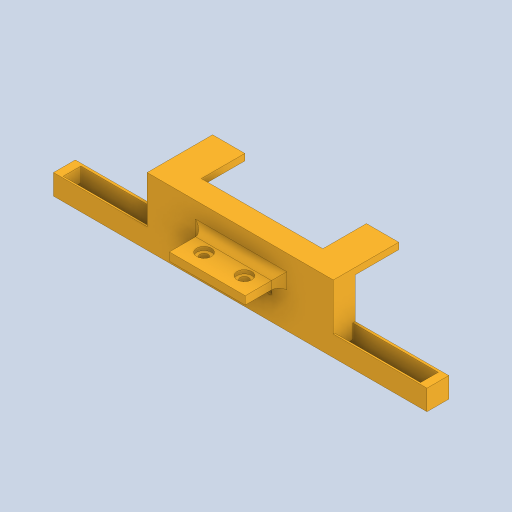
# Autodesk Inventor part: konsept3_med_led_extended
Saved by Autodesk Inventor 2023.1 (Build 271208000, 208)
## iProperties
Created: 2024-07-10
Part Number: konsept3_med_led_extended
Material: S355J2+N
Document SubType Name: Modeling
Designer: huchonms
Engineer: thingelstade
Mass: 592.93 g
Surface Area: 269.172 cm^2
Volume: 75.5325 cm^3
Density: 7.85 g/cm^3
Appearance: Metal (300-500 MPa)
tc_part_rev_length: 231
tc_part_rev_width: 62
tc_part_rev_height: 41.64
tc_part_rev_uom_length: mm
tc_part_rev_volume: 75533
tc_part_rev_uom_volume: mm^3
tc_part_rev_mass: 0.59
tc_part_rev_uom_mass: kg
NOV_FileName: konsept3_med_led_extended
Author: huchonms
Revision Number: 0
Autodesk Inventor part; units mm, degrees
ref_plane "YZ Plane" through (0, 0, 0) normal (1, 0, 0) x (0, 1, 0)
ref_plane "XZ Plane" through (0, 0, 0) normal (0, 1, 0) x (-1, 0, 0)
ref_plane "XY Plane" through (0, 0, 0) normal (0, 0, 1) x (1, 0, 0)
sketch "Sketch1" plane through (0, 0, 0) normal (0, 1, 0) x (-1, 0, 0)
  circle A0 centre (74.3729, -21.8037) radius 1.7645
  circle A1 centre (56.3729, -21.8037) radius 3.0578
  circle A2 centre (38.3729, -21.8037) radius 1.7645
  ellipse E0 centre (18.2576, -20.2741) end of major axis (25.2624, -10.1128) minor radius 8.7701 (8.7502, -27.1013) -> (10.9663, -30.2256) ccw
  spline S0 degree 3 poles (10.9663, -30.2256) (11.558, -30.6853) (12.2409, -31.0443) (12.9908, -31.2838) (13.7407, -31.5232) (14.557, -31.6429) (15.405, -31.6429) knots 0 0 0 0 0.499989 0.499989 0.499989 1 1 1 1
  line L0 (15.405, -31.6429) -> (97.3407, -31.6429)
  spline S1 degree 3 poles (97.3407, -31.6429) (98.1082, -31.6429) (98.8584, -31.5451) (99.5616, -31.3425) (100.2492, -31.1443) (100.8915, -30.8461) (101.4652, -30.4546) (102.0389, -30.063) (102.5439, -29.5783) (102.9657, -29.0193) (103.3971, -28.4476) (103.7414, -27.7985) (103.9955, -27.1013) knots 2.676287 2.676287 2.676287 2.676287 2.891386 2.891386 2.891386 3.101723 3.101723 3.101723 3.312059 3.312059 3.312059 3.527157 3.527157 3.527157 3.527157
  line L1 (103.9955, -27.1013) -> (111.6432, -6.1177)
  spline S2 degree 3 poles (111.6432, -6.1177) (111.7397, -5.8528) (111.8344, -5.5944) (112.022, -5.0857) (112.1147, -4.8357) (112.3029, -4.3319) (112.398, -4.0794) (112.5844, -3.5887) (112.6755, -3.351) (112.8621, -2.8692) (112.9568, -2.6278) (113.1123, -2.2368) (113.1754, -2.0801) (113.2982, -1.7787) (113.3578, -1.6344) (113.4677, -1.3725) (113.5183, -1.2539) (113.6125, -1.0372) (113.6562, -0.9386) (113.7358, -0.763) (113.772, -0.685) (113.8392, -0.544) (113.8704, -0.4806) (113.9275, -0.3682) (113.9537, -0.3186) (113.9875, -0.2575) (113.9966, -0.2414) (114.0055, -0.226) knots 5.498338 5.498338 5.498338 5.498338 5.552114 5.552114 5.607126 5.607126 5.666519 5.666519 5.727103 5.727103 5.795218 5.795218 5.844696 5.844696 5.895721 5.895721 5.943374 5.943374 5.988975 5.988975 6.031119 6.031119 6.071863 6.071863 6.110843 6.110843 6.125778 6.125778 6.125778 6.125778
  spline S3 degree 3 poles (114.0055, -0.226) (113.9928, -0.2026) (113.9622, -0.1742) (113.9104, -0.1385) (113.906, -0.1355) (113.8757, -0.1152) (113.8463, -0.0979) (113.8052, -0.0766) (113.7959, -0.0719) (113.691, -0.0221) (113.6027, 0) (113.5195, 0) knots 0 0 0 0 0.234375 0.234375 0.25 0.25 0.4375 0.4375 0.5 0.5 0.999999 0.999999 0.999999 0.999999
  line L2 (112.7702, 0) -> (113.5195, 0)
  line L3 (112.7702, 0) -> (112.7455, 0)
  line L4 (0, 0) -> (112.7455, 0)
  line L5 (0, 0) -> (-0.0247, 0)
  line L6 (-0.7737, 0) -> (-0.0247, 0)
  spline S4 degree 3 poles (-0.7737, 0) (-0.846, 0) (-0.9227, -0.017) (-1.0154, -0.0558) (-1.0288, -0.0618) (-1.0767, -0.0844) (-1.1139, -0.1052) (-1.153, -0.1307) (-1.1545, -0.1317) (-1.2121, -0.1699) (-1.246, -0.2006) (-1.2597, -0.226) knots 0.000001 0.000001 0.000001 0.000001 0.4375 0.4375 0.5 0.5 0.734375 0.734375 0.75 0.75 1 1 1 1
  spline S5 degree 3 poles (-1.2597, -0.226) (-1.2124, -0.3083) (-1.1576, -0.413) (-1.0955, -0.5406) (-0.951, -0.8374) (-0.7663, -1.2588) (-0.545, -1.7976) (-0.5269, -1.8415) (-0.5086, -1.8863) (-0.4901, -1.9318) (-0.0669, -2.9705) (0.4808, -4.4117) (1.1025, -6.1177) knots 3.299 3.299 3.299 3.299 3.378966 3.378966 3.378966 3.564913 3.564913 3.564913 3.580082 3.580082 3.580082 3.92644 3.92644 3.92644 3.92644
  line L7 (1.1025, -6.1177) -> (8.7502, -27.1013)
  circle A3 centre (56.3729, -21.8037) radius 3.0578
  circle A4 centre (38.3729, -21.8037) radius 1.7645
  circle A5 centre (74.3729, -21.8037) radius 1.7645
  point P0 (47.4044, 14.458)
  constraints: 16 end point, 6 centre point, 17 other
extrude "Extrusion1" add sketch "Sketch1" along normal blind 7.5
sketch "Sketch3" plane through (0, 0, 0) normal (0, 1, 0) x (-1, 0, 0)
  line L0 (32.2898, -10.7134) -> (79.2898, -10.7134)
  line L1 (79.2898, -10.7134) -> (79.2898, -15.7134)
  line L2 (79.2898, -15.7134) -> (32.2898, -15.7134)
  line L3 (32.2898, -15.7134) -> (32.2898, -10.7134)
  point P0 (0, 0)
  constraints: 8 end point, 2 parallel, 1 horizontal, 1 perpendicular
extrude "Extrusion2" add sketch "Sketch3" against normal blind 21
sketch "Sketch4" plane through (0, 0, 0) normal (0, -1, 0) x (1, 0, 0)
  circle A0 centre (-56.3729, -21.8037) radius 3.0578 projected
  circle A1 centre (-56.3729, -21.8037) radius 6.1
  point P0 (0, 0)
  dimension "d6" = 12.2
  constraints: 1 centre point, 1 coincident
  measures "d6" diameter of A1
extrude "Extrusion3" cut sketch "Sketch4" against normal blind 3.5
sketch "Sketch5" plane through (0, 7.5, 0) normal (0, 1, 0) x (1, 0, 0)
  spline S0 degree 3 poles (1.2597, 0.226) (1.2124, 0.3083) (1.1576, 0.413) (1.0955, 0.5406) (0.951, 0.8374) (0.7663, 1.2588) (0.545, 1.7976) (0.5269, 1.8415) (0.5086, 1.8863) (0.4901, 1.9318) (0.0669, 2.9705) (-0.4808, 4.4117) (-1.1025, 6.1177) knots 0 0 0 0 0.127447 0.127447 0.127447 0.423807 0.423807 0.423807 0.447982 0.447982 0.447982 1 1 1 1 projected
  line L0 (-1.1025, 6.1177) -> (-8.7502, 27.1013) projected
  ellipse E0 centre (-18.2576, 20.2741) end of major axis (-25.2624, 10.1128) minor radius 8.7701 (-8.7502, 27.1013) -> (-10.9663, 30.2256) ccw projected
  spline S1 degree 3 poles (-10.9663, 30.2256) (-11.558, 30.6853) (-12.2409, 31.0443) (-12.9908, 31.2838) (-13.7407, 31.5232) (-14.557, 31.6429) (-15.405, 31.6429) knots 0 0 0 0 0.499989 0.499989 0.499989 1 1 1 1 projected
  line L1 (-15.405, 31.6429) -> (-97.3407, 31.6429) projected
  spline S2 degree 3 poles (-97.3407, 31.6429) (-98.1082, 31.6429) (-98.8584, 31.5451) (-99.5616, 31.3425) (-100.2492, 31.1443) (-100.8915, 30.8461) (-101.4652, 30.4546) (-102.0389, 30.063) (-102.5439, 29.5783) (-102.9657, 29.0193) (-103.3971, 28.4476) (-103.7414, 27.7985) (-103.9955, 27.1013) knots 0 0 0 0 0.252799 0.252799 0.252799 0.500001 0.500001 0.500001 0.747202 0.747202 0.747202 1 1 1 1 projected
  line L2 (-103.9955, 27.1013) -> (-111.6432, 6.1177) projected
  spline S3 degree 3 poles (-111.6432, 6.1177) (-111.7397, 5.8528) (-111.8344, 5.5944) (-112.022, 5.0857) (-112.1147, 4.8357) (-112.3029, 4.3319) (-112.398, 4.0794) (-112.5844, 3.5887) (-112.6755, 3.351) (-112.8621, 2.8692) (-112.9568, 2.6278) (-113.1123, 2.2368) (-113.1754, 2.0801) (-113.2982, 1.7787) (-113.3578, 1.6344) (-113.4677, 1.3725) (-113.5183, 1.2539) (-113.6125, 1.0372) (-113.6562, 0.9386) (-113.7358, 0.763) (-113.772, 0.685) (-113.8392, 0.544) (-113.8704, 0.4806) (-113.9275, 0.3682) (-113.9537, 0.3186) (-113.9875, 0.2575) (-113.9966, 0.2414) (-114.0055, 0.226) knots 0 0 0 0 0.085707 0.085707 0.173384 0.173384 0.268043 0.268043 0.364601 0.364601 0.473161 0.473161 0.552018 0.552018 0.633341 0.633341 0.709288 0.709288 0.781966 0.781966 0.849134 0.849134 0.914072 0.914072 0.976197 0.976197 1 1 1 1 projected
  spline S4 degree 3 poles (-114.0055, 0.226) (-113.9928, 0.2026) (-113.9622, 0.1742) (-113.9104, 0.1385) (-113.906, 0.1355) (-113.8757, 0.1152) (-113.8463, 0.0979) (-113.8052, 0.0766) (-113.7959, 0.0719) (-113.691, 0.0221) (-113.6027, 0) (-113.5195, 0) knots 0 0 0 0 0.234375 0.234375 0.25 0.25 0.4375 0.4375 0.5 0.5 1 1 1 1 projected
  line L3 (-113.5195, 0) -> (0.7737, 0) projected
  spline S5 degree 3 poles (0.7737, 0) (0.846, 0) (0.9227, 0.017) (1.0154, 0.0558) (1.0288, 0.0618) (1.0767, 0.0844) (1.1139, 0.1052) (1.153, 0.1307) (1.1545, 0.1317) (1.2121, 0.1699) (1.246, 0.2006) (1.2597, 0.226) knots 0 0 0 0 0.4375 0.4375 0.5 0.5 0.734375 0.734375 0.75 0.75 1 1 1 1 projected
  circle A0 centre (-38.3729, 21.8037) radius 1.7645 projected
  circle A1 centre (-56.3729, 21.8037) radius 3.0578 projected
  circle A2 centre (-74.3729, 21.8037) radius 1.7645 projected
  point P0 (0, 0)
  constraints: 7 other
extrude "Extrusion4" add sketch "Sketch5" along normal blind 3
fillet "Fillet1" radius 4.75 1 edges at (-55.7898, 0, -10.7134)
fillet "Fillet2" radius 4.75 4 edges at (-32.2898, 0, -8.3384) (-32.2898, 0, -13.2134) (-79.2898, 0, -8.3384) (-79.2898, 0, -13.2134)
sketch "Sketch6" plane through (-79.2898, -21, -10.7134) normal (0, 0, 1) x (1, 0, 0)
  circle A0 centre (36, 10.5) radius 2.5
  circle A1 centre (11, 10.5) radius 2.5
  line L0 (0, 16.25) -> (0, 0) projected
  line L1 (47, 16.25) -> (47, 0) projected
  line L2 (47, 0) -> (0, 0) projected
  point P0 (79.2898, 21)
  dimension "d13" = 5
  dimension "d14" = 5
  dimension "d16" = 11
  dimension "d17" = 11
  dimension "d20" = 10.5
  dimension "d21" = 10.5
  constraints: 2 centre point
  measures "d13" diameter of A0
  measures "d14" diameter of A1
  measures "d16" distance from line of L0 A1.centre
  measures "d17" distance from line of L1 A0.centre
  measures "d20" distance from line of L2 A0.centre
  measures "d21" distance from line of L2 A1.centre
extrude "Extrusion5" cut sketch "Sketch6" against normal blind 9
sketch "Sketch7" plane through (-113.5195, 0, 0) normal (0, 0, 1) x (1, 0, 0)
  line L0 (114.7792, 0) -> (114.7792, 10.5) projected
  line L1 (-0.486, 0) -> (-0.486, 10.5) projected
  line L2 (0, 10.5) -> (114.2932, 10.5) projected
  line L3 (-0.486, 10.5) -> (0, 10.5) projected
  line L4 (114.2932, 10.5) -> (114.7792, 10.5) projected
  line L5 (0, 0) -> (114.2932, 0) projected
  line L6 (114.2932, 0) -> (114.7792, 0) projected
  line L7 (-0.486, 0) -> (0, 0) projected
  point P0 (113.5195, 0)
extrude "Extrusion6" add sketch "Sketch7" along normal blind 2
sketch "Sketch8" plane through (0, 10.5, 0) normal (0, 1, 0) x (1, 0, 0)
  line L0 (1.2597, -2) -> (-114.0055, -2) projected
  line L1 (1.2597, 0) -> (1.2597, -2) projected
  line L2 (-114.0055, 0) -> (-114.0055, -2) projected
  line L3 (1.2597, 0) -> (-114.0055, 0)
  point P0 (0, 0)
  constraints: 2 end point, 1 horizontal
extrude "Extrusion7" add sketch "Sketch8" along normal blind 3
sketch "Sketch9" plane through (0, 0, 0) normal (0, -1, 0) x (1, 0, 0)
  line L0 (0.7737, 0) -> (1.2597, 0) projected
  spline S0 degree 3 poles (0.7737, 0) (0.846, 0) (0.9227, -0.017) (1.0154, -0.0558) (1.0288, -0.0618) (1.0767, -0.0844) (1.1139, -0.1052) (1.153, -0.1307) (1.1545, -0.1317) (1.2121, -0.1699) (1.246, -0.2006) (1.2597, -0.226) knots 0 0 0 0 0.4375 0.4375 0.5 0.5 0.734375 0.734375 0.75 0.75 1 1 1 1 projected
  line L1 (1.2597, -0.226) -> (1.2597, 0)
  point P0 (0, 0)
  constraints: 2 end point, 1 vertical, 1 other
extrude "Extrusion8" add sketch "Sketch9" against normal up to surface (10.5 mm away)
sketch "Sketch10" plane through (0, 0, 0) normal (0, -1, 0) x (1, 0, 0)
  line L0 (-114.0055, 0) -> (-113.5195, 0) projected
  spline S0 degree 3 poles (-114.0055, -0.226) (-113.9928, -0.2026) (-113.9622, -0.1742) (-113.9104, -0.1385) (-113.906, -0.1355) (-113.8757, -0.1152) (-113.8463, -0.0979) (-113.8052, -0.0766) (-113.7959, -0.0719) (-113.691, -0.0221) (-113.6027, 0) (-113.5195, 0) knots 0 0 0 0 0.234375 0.234375 0.25 0.25 0.4375 0.4375 0.5 0.5 1 1 1 1 projected
  line L1 (-114.0055, -0.226) -> (-114.0055, 0)
  point P0 (0, 0)
  constraints: 2 end point, 1 vertical, 1 other
extrude "Extrusion9" add sketch "Sketch10" against normal up to surface (10.5 mm away)
sketch "Sketch11" plane through (0, 13.5, 0) normal (0, 1, 0) x (1, 0, 0)
  line L0 (-114.0055, -2) -> (1.2597, -2) projected
  line L1 (1.2597, -2) -> (1.2597, 0) projected
  line L2 (1.2597, 0) -> (-18.7403, 0)
  line L3 (-18.7403, 0) -> (-18.7403, -4)
  line L4 (-18.7403, -4) -> (1.2597, -4)
  line L5 (1.2597, -4) -> (1.2597, 0)
  line L6 (-114.0055, 0) -> (-94.0055, 0)
  line L7 (-94.0055, 0) -> (-94.0055, -4)
  line L8 (-94.0055, -4) -> (-114.0055, -4)
  line L9 (-114.0055, -4) -> (-114.0055, 0)
  point P0 (0, 0)
  dimension "d30" = 20
  dimension "d31" = 20
  constraints: 16 end point, 4 parallel, 2 horizontal, 2 perpendicular, 2 point on line
  measures "d30" distance of L4.end L3.end
  measures "d31" distance of L7.end L8.end
extrude "Extrusion10" add sketch "Sketch11" along normal blind 14
sketch "Sketch12" plane through (0, 13.5, 0) normal (0, 1, 0) x (1, 0, 0)
  line L0 (-18.7403, -2) -> (-18.7403, 0) projected
  line L1 (-94.0055, -2) -> (-18.7403, -2) projected
  line L2 (-18.7403, 0) -> (-94.0055, 0) projected
  line L3 (-94.0055, 0) -> (-94.0055, -2) projected
  point P0 (0, 0)
extrude "Extrusion11" cut sketch "Sketch12" against normal up to surface (3 mm away)
sketch "Sketch13" plane through (0, 13.5, 0) normal (0, -1, 0) x (1, 0, 0)
  line L0 (-114.0055, 2) -> (-94.0055, 2) projected
  line L1 (-94.0055, 4) -> (-94.0055, 2) projected
  line L2 (-114.0055, 4) -> (-94.0055, 4) projected
  line L3 (-114.0055, 2) -> (-114.0055, 4) projected
  line L4 (-18.7403, 2) -> (1.2597, 2) projected
  line L5 (1.2597, 4) -> (1.2597, 2) projected
  line L6 (-18.7403, 4) -> (1.2597, 4) projected
  line L7 (-18.7403, 2) -> (-18.7403, 4) projected
  point P0 (0, 0)
extrude "Extrusion12" add sketch "Sketch13" along normal up to surface (13.5 mm away)
sketch "Sketch14" plane through (-94.0055, 0, 4) normal (1, 0, 0) x (0, 0, -1)
  line L0 (2, 10.5) -> (2, 0) projected
  line L1 (2, 0) -> (0, 0) projected
  line L2 (0, 27.5) -> (0, 0) projected
  line L3 (2, 10.5) -> (0, 10.5)
  point P0 (4, 0)
  constraints: 2 end point, 1 perpendicular, 1 point on line
extrude "Extrusion13" add sketch "Sketch14" along normal up to surface (75.2652 mm away)
sketch "Sketch15" plane through (-114.0055, 0, 4) normal (0, 0, 1) x (1, 0, 0)
  circle A0 centre (105.2652, 19) radius 4.5
  circle A1 centre (10, 19) radius 4.5
  line L0 (95.2652, 10.5) -> (95.2652, 27.5) projected
  line L1 (0, 0) -> (0, 27.5) projected
  line L2 (95.2652, 27.5) -> (115.2652, 27.5) projected
  line L3 (0, 27.5) -> (20, 27.5) projected
  point P0 (114.0055, 0)
  dimension "d40" = 9
  dimension "d41" = 9
  dimension "d42" = 10
  dimension "d43" = 10
  dimension "d44" = 8.5
  dimension "d45" = 8.5
  constraints: 2 centre point
  measures "d40" diameter of A0
  measures "d41" diameter of A1
  measures "d42" distance from line of L0 A0.centre
  measures "d43" distance from line of L1 A1.centre
  measures "d44" distance from line of L2 A0.centre
  measures "d45" distance from line of L3 A1.centre
extrude "Extrusion14" cut sketch "Sketch15" against normal blind 2.2
sketch "Sketch16" plane through (-8.7403, 19, 1.8) normal (0, 0, 1) x (1, 0, 0)
  circle A0 centre (0, 0) radius 2.5
  circle A1 centre (-95, 0) radius 2.5
  point P0 (8.7403, -19)
  dimension "d48" = 5
  dimension "d49" = 5
  constraints: 2 centre point
  measures "d48" diameter of A0
  measures "d49" diameter of A1
extrude "Extrusion15" cut sketch "Sketch16" against normal blind 4.05
thread "Thread1" size "M5x0.8" designation "M5" standard "Metric Standard" full length
thread "Thread2" size "M5x0.8" designation "M5" standard "Metric Standard" full length
sketch "Sketch18" plane through (-8.7403, 19, 0) normal (1, 0, 0) x (0, 1, 0)
  line L0 (2.5, 0) -> (2.5, 1.8)
  line L1 (2.5, 1.8) -> (1.9068, 1.8)
  line L2 (1.9068, 1.8) -> (1.9068, 0)
  line L3 (1.9068, 0) -> (2.5, 0)
  line L4 (0, -38.7715) -> (0, 11.1286) projected
  constraints: 8 end point
revolve "Revolution1" add sketch "Sketch18" angle 360 about axis through (-8.7403, 19, 0) along (0, 0, 1) separate body
sketch "Sketch17" plane through (-8.7403, 21.5, 0) normal (-1, 0, 0) x (0, 0, 1)
  line L0 (-0.4668, -0.0406) -> (-0.4001, -0.0406) construction
  line L1 (0.0666, -0.5529) -> (-0.0001, -0.6809) construction
  line L2 (-0.8001, -0.6809) -> (-0.8668, -0.5529) construction
  line L3 (-0.3334, -0.0406) -> (-0.4001, 0.0874) construction
  line L4 (-0.4001, 0.0874) -> (-0.4668, -0.0406) construction
  line L5 (-0.8001, -0.6809) -> (-0.7334, -0.5529) construction
  line L6 (-0.3334, -0.0406) -> (-0.0668, -0.5529)
  line L7 (-0.8668, -0.5529) -> (-0.7334, -0.5529) construction
  arc A0 (-0.8668, -0.5529) -> (-0.8001, -0.5933) centre (-0.8001, -0.5182) ccw construction
  line L8 (0.0666, -0.5529) -> (-0.0668, -0.5529) construction
  line L9 (-0.8001, -0.6809) -> (-0.8001, -0.5529) construction
  line L10 (-0.0001, -0.6809) -> (-0.0001, -0.5529) construction
  line L11 (-0.4001, 0.0874) -> (-0.4001, -0.0002) construction
  line L12 (-0.8001, -0.5933) -> (-0.0001, -0.5933)
  arc A1 (-0.8001, -0.5933) -> (-0.7334, -0.5529) centre (-0.8001, -0.5182) ccw
  line L13 (-0.0668, -0.5529) -> (-0.0001, -0.6809) construction
  line L14 (-0.7334, -0.5529) -> (-0.4668, -0.0406)
  line L15 (-0.0001, -0.0002) -> (-0.0001, 0.0177)
  line L16 (-0.0001, 0.0177) -> (-0.0001, -0.0002)
  line L17 (-0.0001, -0.0002) -> (0.0334, -0.0002)
  arc A2 (-0.0668, -0.5529) -> (-0.0001, -0.5933) centre (-0.0001, -0.5182) ccw
  arc A3 (-0.0001, -0.5933) -> (0.0666, -0.5529) centre (-0.0001, -0.5182) ccw construction
  arc A4 (-0.4001, -0.0002) -> (-0.4668, -0.0406) centre (-0.4001, -0.0753) ccw
  arc A5 (-0.3334, -0.0406) -> (-0.4001, -0.0002) centre (-0.4001, -0.0753) ccw
  line L18 (-0.4001, -0.0002) -> (-0.4001, -0.0406) construction
  line L19 (-0.4001, -0.0406) -> (-0.3334, -0.0406) construction
  dimension "d56" = 55
  dimension "d57" = 0.1281
  dimension "d58" = 0.1281
  dimension "Sketch17_ThreadOffset" = 0
  dimension "Sketch17_MajorRadius" = 0.5932
  dimension "d61" = 0.8
  dimension "Sketch17_MinorRadius" = 0
  constraints: 40 end point, 12 point on circle, 10 parallel, 8 tangent, 6 centre point, 6 collinear, 2 midpoint, 2 point on line, 1 horizontal, 1 perpendicular, 3 other
  measures "d56" angle of L6 L14
  measures "d57" distance of L3.end L0.end
  measures "d58" distance of L1.end L10.end
  measures "Sketch17_ThreadOffset" distance between parallel lines of L15 L10
  measures "Sketch17_MajorRadius" distance from line of L12 L15.start
  measures "d61" distance from line of L1.end L9
  measures "Sketch17_MinorRadius" distance edge to line of A5 L17
coil "Coil1" sketch "Sketch17" operation cut axis through (-8.7403, 19, 0) along (0, 0, 1) pitch 0.8008 turns 4.245754 hand right bodies 2
sketch "Sketch20" plane through (-103.7403, 19, 0) normal (1, 0, 0) x (0, 1, 0)
  line L0 (2.5, 0) -> (2.5, 1.8)
  line L1 (2.5, 1.8) -> (1.9068, 1.8)
  line L2 (1.9068, 1.8) -> (1.9068, 0)
  line L3 (1.9068, 0) -> (2.5, 0)
  line L4 (0, -38.7715) -> (0, 11.1286) projected
  constraints: 8 end point
revolve "Revolution2" add sketch "Sketch20" angle 360 about axis through (-103.7403, 19, 0) along (0, 0, 1) separate body
sketch "Sketch19" plane through (-103.7403, 21.5, 0) normal (-1, 0, 0) x (0, 0, 1)
  line L0 (-0.4668, -0.0406) -> (-0.4001, -0.0406) construction
  line L1 (0.0666, -0.5529) -> (-0.0001, -0.6809) construction
  line L2 (-0.8001, -0.6809) -> (-0.8668, -0.5529) construction
  line L3 (-0.3334, -0.0406) -> (-0.4001, 0.0874) construction
  line L4 (-0.4001, 0.0874) -> (-0.4668, -0.0406) construction
  line L5 (-0.8001, -0.6809) -> (-0.7334, -0.5529) construction
  line L6 (-0.3334, -0.0406) -> (-0.0668, -0.5529)
  line L7 (-0.8668, -0.5529) -> (-0.7334, -0.5529) construction
  arc A0 (-0.8668, -0.5529) -> (-0.8001, -0.5933) centre (-0.8001, -0.5182) ccw construction
  line L8 (0.0666, -0.5529) -> (-0.0668, -0.5529) construction
  line L9 (-0.8001, -0.6809) -> (-0.8001, -0.5529) construction
  line L10 (-0.0001, -0.6809) -> (-0.0001, -0.5529) construction
  line L11 (-0.4001, 0.0874) -> (-0.4001, -0.0002) construction
  line L12 (-0.8001, -0.5933) -> (-0.0001, -0.5933)
  arc A1 (-0.8001, -0.5933) -> (-0.7334, -0.5529) centre (-0.8001, -0.5182) ccw
  line L13 (-0.0668, -0.5529) -> (-0.0001, -0.6809) construction
  line L14 (-0.7334, -0.5529) -> (-0.4668, -0.0406)
  line L15 (-0.0001, -0.0002) -> (-0.0001, 0.0177)
  line L16 (-0.0001, 0.0177) -> (-0.0001, -0.0002)
  line L17 (-0.0001, -0.0002) -> (0.0334, -0.0002)
  arc A2 (-0.0668, -0.5529) -> (-0.0001, -0.5933) centre (-0.0001, -0.5182) ccw
  arc A3 (-0.0001, -0.5933) -> (0.0666, -0.5529) centre (-0.0001, -0.5182) ccw construction
  arc A4 (-0.4001, -0.0002) -> (-0.4668, -0.0406) centre (-0.4001, -0.0753) ccw
  arc A5 (-0.3334, -0.0406) -> (-0.4001, -0.0002) centre (-0.4001, -0.0753) ccw
  line L18 (-0.4001, -0.0002) -> (-0.4001, -0.0406) construction
  line L19 (-0.4001, -0.0406) -> (-0.3334, -0.0406) construction
  dimension "d74" = 55
  dimension "d75" = 0.1281
  dimension "d76" = 0.1281
  dimension "Sketch19_ThreadOffset" = 0
  dimension "Sketch19_MajorRadius" = 0.5932
  dimension "d79" = 0.8
  dimension "Sketch19_MinorRadius" = 0
  constraints: 40 end point, 12 point on circle, 10 parallel, 8 tangent, 6 centre point, 6 collinear, 2 midpoint, 2 point on line, 1 horizontal, 1 perpendicular, 3 other
  measures "d74" angle of L6 L14
  measures "d75" distance of L3.end L0.end
  measures "d76" distance of L1.end L10.end
  measures "Sketch19_ThreadOffset" distance between parallel lines of L15 L10
  measures "Sketch19_MajorRadius" distance from line of L12 L15.start
  measures "d79" distance from line of L1.end L9
  measures "Sketch19_MinorRadius" distance edge to line of A5 L17
coil "Coil2" sketch "Sketch19" operation cut axis through (-103.7403, 19, 0) along (0, 0, 1) pitch 0.8008 turns 4.245754 hand right bodies 3
sketch "Sketch21" plane through (-114.0055, 0, 4) normal (0, 0, 1) x (1, 0, 0)
  circle A0 centre (105.2652, 19) radius 4.5 projected
  circle A1 centre (10, 19) radius 4.5 projected
  point P0 (114.0055, 0)
extrude "Extrusion16" add sketch "Sketch21" against normal up to surface (4 mm away) bodies 1
sketch "Sketch22" plane through (0, 27.5, 0) normal (0, 1, 0) x (1, 0, 0)
  line L0 (-18.7403, 0) -> (-18.7403, -4) projected
  line L1 (-18.7403, -4) -> (1.2597, -4) projected
  line L2 (1.2597, -4) -> (1.2597, 0) projected
  line L3 (1.2597, 0) -> (-18.7403, 0) projected
  line L4 (-94.0055, -4) -> (-94.0055, 0) projected
  line L5 (-94.0055, 0) -> (-114.0055, 0) projected
  line L6 (-114.0055, 0) -> (-114.0055, -4) projected
  line L7 (-114.0055, -4) -> (-94.0055, -4) projected
  point P0 (0, 0)
extrude "Extrusion17" add sketch "Sketch22" along normal blind 13 bodies 1
sketch "Sketch23" plane through (-114.0055, 0, 4) normal (0, 0, 1) x (1, 0, 0)
  point P0 (114.0055, 0)
sketch "Sketch24" plane through (0, 10.5, 0) normal (0, 1, 0) x (1, 0, 0)
  line L0 (1.2597, 0) -> (-18.7403, 0) projected
  line L1 (1.2597, 0.226) -> (1.2597, 0) projected
  spline S0 degree 3 poles (1.2597, 0.226) (1.2124, 0.3083) (1.1576, 0.413) (1.0955, 0.5406) (0.951, 0.8374) (0.7663, 1.2588) (0.545, 1.7976) (0.5269, 1.8415) (0.5086, 1.8863) (0.4901, 1.9318) (0.0669, 2.9705) (-0.4808, 4.4117) (-1.1025, 6.1177) knots 0 0 0 0 0.127447 0.127447 0.127447 0.423807 0.423807 0.423807 0.447982 0.447982 0.447982 1 1 1 1 projected
  line L2 (-1.1025, 6.1177) -> (-8.7502, 27.1013) projected
  ellipse E0 centre (-18.2576, 20.2741) end of major axis (-25.2624, 10.1128) minor radius 8.7701 (-8.7502, 27.1013) -> (-10.9663, 30.2256) ccw projected
  spline S1 degree 3 poles (-10.9663, 30.2256) (-11.558, 30.6853) (-12.2409, 31.0443) (-12.9908, 31.2838) (-13.7407, 31.5232) (-14.557, 31.6429) (-15.405, 31.6429) knots 0 0 0 0 0.499989 0.499989 0.499989 1 1 1 1 projected
  line L3 (-15.405, 31.6429) -> (-97.3407, 31.6429) projected
  spline S2 degree 3 poles (-97.3407, 31.6429) (-98.1082, 31.6429) (-98.8584, 31.5451) (-99.5616, 31.3425) (-100.2492, 31.1443) (-100.8915, 30.8461) (-101.4652, 30.4546) (-102.0389, 30.063) (-102.5439, 29.5783) (-102.9657, 29.0193) (-103.3971, 28.4476) (-103.7414, 27.7985) (-103.9955, 27.1013) knots 0 0 0 0 0.252799 0.252799 0.252799 0.500001 0.500001 0.500001 0.747202 0.747202 0.747202 1 1 1 1 projected
  line L4 (-103.9955, 27.1013) -> (-111.6432, 6.1177) projected
  spline S3 degree 3 poles (-111.6432, 6.1177) (-111.7397, 5.8528) (-111.8344, 5.5944) (-112.022, 5.0857) (-112.1147, 4.8357) (-112.3029, 4.3319) (-112.398, 4.0794) (-112.5844, 3.5887) (-112.6755, 3.351) (-112.8621, 2.8692) (-112.9568, 2.6278) (-113.1123, 2.2368) (-113.1754, 2.0801) (-113.2982, 1.7787) (-113.3578, 1.6344) (-113.4677, 1.3725) (-113.5183, 1.2539) (-113.6125, 1.0372) (-113.6562, 0.9386) (-113.7358, 0.763) (-113.772, 0.685) (-113.8392, 0.544) (-113.8704, 0.4806) (-113.9275, 0.3682) (-113.9537, 0.3186) (-113.9875, 0.2575) (-113.9966, 0.2414) (-114.0055, 0.226) knots 0 0 0 0 0.085707 0.085707 0.173384 0.173384 0.268043 0.268043 0.364601 0.364601 0.473161 0.473161 0.552018 0.552018 0.633341 0.633341 0.709288 0.709288 0.781966 0.781966 0.849134 0.849134 0.914072 0.914072 0.976197 0.976197 1 1 1 1 projected
  line L5 (-114.0055, 0) -> (-114.0055, 0.226) projected
  line L6 (-94.0055, 0) -> (-114.0055, 0) projected
  line L7 (-94.0055, -4) -> (-94.0055, 0) projected
  line L8 (-94.0055, -4) -> (-18.7403, -4) projected
  line L9 (-18.7403, 0) -> (-18.7403, -4) projected
  circle A0 centre (-38.3729, 21.8037) radius 1.7645 projected
  circle A1 centre (-56.3729, 21.8037) radius 3.0578 projected
  circle A2 centre (-74.3729, 21.8037) radius 1.7645 projected
  point P0 (0, 0)
  constraints: 5 other
extrude "Extrusion18" add sketch "Sketch24" along normal blind 3 bodies 1
sketch "Sketch25" plane through (-114.0055, 0, 4) normal (0, 0, 1) x (1, 0, 0)
  point P0 (114.0055, 0)
sketch "Sketch26" plane through (0, 0, 0) normal (0, -1, 0) x (1, 0, 0)
  line L0 (-15.405, -31.6429) -> (-97.3407, -31.6429) projected
  line L1 (1.2597, 4) -> (-114.0055, 4) projected
  line L2 (-97.3407, -31.6429) -> (-114.0055, -31.6429)
  line L3 (-114.0055, -31.6429) -> (-114.0055, 4)
  spline S0 degree 3 poles (-97.3407, -31.6429) (-98.1082, -31.6429) (-98.8584, -31.5451) (-99.5616, -31.3425) (-100.2492, -31.1443) (-100.8915, -30.8461) (-101.4652, -30.4546) (-102.0389, -30.063) (-102.5439, -29.5783) (-102.9657, -29.0193) (-103.3971, -28.4476) (-103.7414, -27.7985) (-103.9955, -27.1013) knots 0 0 0 0 0.252799 0.252799 0.252799 0.500001 0.500001 0.500001 0.747202 0.747202 0.747202 1 1 1 1 projected
  line L4 (-103.9955, -27.1013) -> (-111.6432, -6.1177) projected
  spline S1 degree 3 poles (-111.6432, -6.1177) (-111.7397, -5.8528) (-111.8344, -5.5944) (-112.022, -5.0857) (-112.1147, -4.8357) (-112.3029, -4.3319) (-112.398, -4.0794) (-112.5844, -3.5887) (-112.6755, -3.351) (-112.8621, -2.8692) (-112.9568, -2.6278) (-113.1123, -2.2368) (-113.1754, -2.0801) (-113.2982, -1.7787) (-113.3578, -1.6344) (-113.4677, -1.3725) (-113.5183, -1.2539) (-113.6125, -1.0372) (-113.6562, -0.9386) (-113.7358, -0.763) (-113.772, -0.685) (-113.8392, -0.544) (-113.8704, -0.4806) (-113.9275, -0.3682) (-113.9537, -0.3186) (-113.9875, -0.2575) (-113.9966, -0.2414) (-114.0055, -0.226) knots 0 0 0 0 0.085707 0.085707 0.173384 0.173384 0.268043 0.268043 0.364601 0.364601 0.473161 0.473161 0.552018 0.552018 0.633341 0.633341 0.709288 0.709288 0.781966 0.781966 0.849134 0.849134 0.914072 0.914072 0.976197 0.976197 1 1 1 1 projected
  point P0 (0, 0)
  constraints: 4 end point, 1 horizontal, 1 perpendicular, 2 other
extrude "Extrusion19" add sketch "Sketch26" against normal up to surface (13.5 mm away) bodies 1
sketch "Sketch27" plane through (0, 13.5, 0) normal (0, 1, 0) x (1, 0, 0)
  spline S0 degree 3 poles (-10.9663, 30.2256) (-11.558, 30.6853) (-12.2409, 31.0443) (-12.9908, 31.2838) (-13.7407, 31.5232) (-14.557, 31.6429) (-15.405, 31.6429) knots 0 0 0 0 0.499989 0.499989 0.499989 1 1 1 1 projected
  ellipse E0 centre (-18.2576, 20.2741) end of major axis (-25.2624, 10.1128) minor radius 8.7701 (-8.7502, 27.1013) -> (-10.9663, 30.2256) ccw projected
  line L0 (-1.1025, 6.1177) -> (-8.7502, 27.1013) projected
  spline S1 degree 3 poles (1.2597, 0.226) (1.2124, 0.3083) (1.1576, 0.413) (1.0955, 0.5406) (0.951, 0.8374) (0.7663, 1.2588) (0.545, 1.7976) (0.5269, 1.8415) (0.5086, 1.8863) (0.4901, 1.9318) (0.0669, 2.9705) (-0.4808, 4.4117) (-1.1025, 6.1177) knots 0 0 0 0 0.127447 0.127447 0.127447 0.423807 0.423807 0.423807 0.447982 0.447982 0.447982 1 1 1 1 projected
  line L1 (-15.405, 31.6429) -> (1.2597, 31.6429)
  line L2 (1.2597, 31.6429) -> (1.2597, 0.226)
  point P0 (0, 0)
  constraints: 4 end point, 1 horizontal, 1 perpendicular, 3 other
extrude "Extrusion20" add sketch "Sketch27" against normal up to surface (13.5 mm away) bodies 1
sketch "Sketch28" plane through (1.2597, 0, 4) normal (1, 0, 0) x (0, 0, -1)
  line L0 (35.6429, 13.5) -> (35.6429, 0) projected
  line L1 (4, 13.5) -> (35.6429, 13.5) projected
  line L2 (35.6429, 0) -> (0, 0) projected
  line L3 (29, 0) -> (29, 13.5)
  point P0 (4, 0)
  constraints: 2 end point, 2 point on line, 1 perpendicular
extrude "Extrusion21" add sketch "Sketch28" along normal blind 70 bodies 1
sketch "Sketch29" plane through (-114.0055, 0, -31.6429) normal (-1, 0, 0) x (0, 0, 1)
  line L0 (0, 13.5) -> (6.6429, 13.5) projected
  line L1 (6.6429, 13.5) -> (6.6429, 0) projected
  line L2 (6.6429, 0) -> (0, 0) projected
  line L3 (0, 0) -> (0, 13.5) projected
  point P0 (31.6429, 0)
extrude "Extrusion22" add sketch "Sketch29" along normal blind 70 bodies 1
sketch "Sketch30" plane through (1.2597, 0, -25) normal (0, 0, 1) x (1, 0, 0)
  point P0 (-1.2597, 0)
sketch "Sketch31" plane through (1.2597, 0, -25) normal (0, 0, 1) x (1, 0, 0)
  line L0 (67, 12) -> (-16, 12)
  line L1 (-16, 12) -> (-16, 1)
  line L2 (-16, 1) -> (67, 1)
  line L3 (67, 1) -> (67, 12)
  line L4 (67, 12) -> (-16, 1) construction
  line L5 (-16, 12) -> (67, 1) construction
  line L6 (70, 13.5) -> (70, 0) projected
  point P0 (-1.2597, 0)
  point P1 (25.5, 6.5)
  dimension "d106" = 83
  dimension "d107" = 11
  dimension "d108" = 3
  constraints: 12 end point, 2 midpoint, 2 parallel, 1 horizontal, 1 perpendicular
  measures "d106" distance of L1.end L2.end
  measures "d107" distance of L2.end L0.start
  measures "d108" distance between parallel lines of L6 L3
sketch "Sketch32" plane through (-114.0055, 0, -25) normal (0, 0, 1) x (1, 0, 0)
  line L0 (16, 0.9533) -> (-67, 0.9533)
  line L1 (-67, 0.9533) -> (-67, 11.9533)
  line L2 (-67, 11.9533) -> (16, 11.9533)
  line L3 (16, 11.9533) -> (16, 0.9533)
  line L4 (16, 0.9533) -> (-67, 11.9533) construction
  line L5 (-67, 0.9533) -> (16, 11.9533) construction
  line L6 (-70, 0) -> (-70, 13.5) projected
  point P0 (114.0055, 0)
  point P1 (-25.5, 6.4533)
  dimension "d109" = 83
  dimension "d110" = 11
  dimension "d111" = 3
  constraints: 12 end point, 2 midpoint, 2 parallel, 1 horizontal, 1 perpendicular
  measures "d109" distance of L1.end L2.end
  measures "d110" distance of L0.end L1.end
  measures "d111" distance between parallel lines of L6 L1
extrude "Extrusion23" cut sketch "Sketch31" along normal mid plane 70 bodies 1
extrude "Extrusion24" cut sketch "Sketch32" along normal mid plane 70 bodies 1
sketch "Sketch33" plane through (-114.0055, 0, 4) normal (0, 0, 1) x (1, 0, 0)
  line L0 (0, 11.9533) -> (16, 11.9533) projected
  line L1 (16, 11.9533) -> (16, 0.9533) projected
  line L2 (16, 0.9533) -> (0, 0.9533) projected
  line L3 (0, 11.9533) -> (0, 0.9533)
  point P0 (114.0055, 0)
  constraints: 2 end point, 1 vertical
extrude "Extrusion25" add sketch "Sketch33" against normal up to surface (29 mm away) bodies 1
sketch "Sketch34" plane through (-114.0055, 0, 4) normal (0, 0, 1) x (1, 0, 0)
  line L0 (99.2652, 1) -> (99.2652, 12) projected
  line L1 (99.2652, 12) -> (115.2652, 12) projected
  line L2 (115.2652, 1) -> (99.2652, 1) projected
  line L3 (115.2652, 1) -> (115.2652, 12)
  point P0 (114.0055, 0)
  constraints: 2 end point, 1 vertical
extrude "Extrusion26" add sketch "Sketch34" against normal up to surface (29 mm away) bodies 1
sketch "Sketch35" plane through (1.2597, 12, -25) normal (0, 0, -1) x (-1, 0, 0)
  line L0 (99.2652, -11.0467) -> (99.2652, -0.0467) projected
  line L1 (115.2652, -11.0467) -> (99.2652, -11.0467) projected
  line L2 (115.2652, -11.0467) -> (115.2652, -0.0467) projected
  line L3 (99.2652, -0.0467) -> (115.2652, -0.0467) projected
  line L4 (16, 0) -> (16, -11) projected
  line L5 (0, 0) -> (16, 0) projected
  line L6 (0, 0) -> (0, -11) projected
  line L7 (16, -11) -> (0, -11) projected
  point P0 (1.2597, -12)
extrude "Extrusion27" add sketch "Sketch35" along normal blind 3 bodies 1
sketch "Sketch36" plane through (-181.0055, 0.9533, -25) normal (1, 0, 0) x (0, 0, -1)
  line L0 (3, 0) -> (3, 11) projected
  line L1 (0, 0) -> (3, 0) projected
  line L2 (3, 11) -> (0, 11) projected
  line L3 (0, 0) -> (0, 11) projected
  point P0 (-25, -0.9533)
extrude "Extrusion28" add sketch "Sketch36" along normal blind 5.5 bodies 1
sketch "Sketch37" plane through (-98.0055, 0.9533, -31.6429) normal (-1, 0, 0) x (0, 0, 1)
  line L0 (3.6429, 0) -> (3.6429, 11) projected
  line L1 (3.6429, 11) -> (0, 11) projected
  line L2 (0, 0) -> (0, 11) projected
  line L3 (0, 0) -> (3.6429, 0) projected
  point P0 (31.6429, -0.9533)
extrude "Extrusion29" cut sketch "Sketch37" against normal blind 10 bodies 1
sketch "Sketch38" plane through (-181.0055, 0.9533, -31.6429) normal (1, 0, 0) x (0, 0, -1)
  line L0 (-3.6429, 11) -> (-3.6429, 0) projected
  line L1 (0, 0) -> (-3.6429, 0) projected
  line L2 (0, 11) -> (0, 0) projected
  line L3 (0, 11) -> (-3.6429, 11) projected
  point P0 (-31.6429, -0.9533)
extrude "Extrusion30" add sketch "Sketch38" along normal blind 10 bodies 1
sketch "Sketch39" plane through (-175.5055, 0.9533, -25) normal (1, 0, 0) x (0, 0, -1)
  line L0 (3, 0) -> (3, 11) projected
  line L1 (0, 11) -> (3, 11) projected
  line L2 (0, 11) -> (0, 0) projected
  line L3 (3, 0) -> (0, 0) projected
  point P0 (-25, -0.9533)
extrude "Extrusion31" add sketch "Sketch39" along normal up to surface (4.5 mm away) bodies 1
sketch "Sketch40" plane through (68.2597, 1, -25) normal (-1, 0, 0) x (0, 0, 1)
  line L0 (0, 11) -> (0, 0) projected
  line L1 (-6.6429, 11) -> (0, 11) projected
  line L2 (-6.6429, 0) -> (-6.6429, 11) projected
  line L3 (-6.6429, 0) -> (0, 0) projected
  point P0 (25, -1)
extrude "Extrusion32" add sketch "Sketch40" along normal blind 10 bodies 1
sketch "Sketch41" plane through (-14.7403, 1, -31.6429) normal (1, 0, 0) x (0, 0, -1)
  line L0 (-3.6429, 11) -> (-3.6429, 0) projected
  line L1 (0, 0) -> (-3.6429, 0) projected
  line L2 (0, 11) -> (0, 0) projected
  line L3 (-3.6429, 11) -> (0, 11) projected
  point P0 (-31.6429, -1)
extrude "Extrusion33" cut sketch "Sketch41" against normal blind 10 bodies 1
sketch "Sketch42" plane through (71.2597, 0, -31.6429) normal (0, 0, -1) x (-1, 0, 0)
  line L0 (0, 0) -> (0, 13.5) projected
  line L1 (0, 13.5) -> (255.2652, 13.5) projected
  line L2 (255.2652, 0) -> (0, 0) projected
  line L3 (13, 12) -> (13, 1) projected
  line L4 (12, 13.5) -> (12, 0)
  point P0 (71.2597, 0)
  dimension "d134" = 1
  constraints: 2 end point, 2 point on line, 1 perpendicular
  measures "d134" distance between parallel lines of L3 L4
extrude "Extrusion34" cut sketch "Sketch42" against normal blind 9 bodies 1
sketch "Sketch43" plane through (-184.0055, 0, -31.6429) normal (0, 0, -1) x (-1, 0, 0)
  line L0 (-243.2652, 13.5) -> (0, 13.5) projected
  line L1 (0, 13.5) -> (0, 0) projected
  line L2 (0, 0) -> (-243.2652, 0) projected
  line L3 (-13, 0.9533) -> (-13, 11.9533) projected
  line L4 (-12, 13.5) -> (-12, 0)
  point P0 (-184.0055, 0)
  dimension "d137" = 1
  constraints: 2 end point, 2 point on line, 1 perpendicular
  measures "d137" distance between parallel lines of L4 L3
extrude "Extrusion35" cut sketch "Sketch43" against normal blind 17.25 bodies 1
sketch "Sketch44" plane through (-172.0055, 0, -31.6429) normal (-1, 0, 0) x (0, 0, 1)
  line L0 (3.6429, 0.9533) -> (3.6429, 11.9533) projected
  line L1 (6.6429, 0.9533) -> (3.6429, 0.9533) projected
  line L2 (3.6429, 11.9533) -> (6.6429, 11.9533) projected
  line L3 (6.6429, 0.9533) -> (6.6429, 11.9533) projected
  point P0 (31.6429, 0)
extrude "Extrusion36" add sketch "Sketch44" against normal blind 5 bodies 1
sketch "Sketch45" plane through (59.2597, 0, -31.6429) normal (1, 0, 0) x (0, 0, -1)
  line L0 (-3.6429, 1) -> (-6.6429, 1) projected
  line L1 (-3.6429, 12) -> (-3.6429, 1) projected
  line L2 (-6.6429, 12) -> (-3.6429, 12) projected
  line L3 (-6.6429, 0) -> (-6.6429, 13.5) projected
  point P0 (-31.6429, 0)
extrude "Extrusion37" add sketch "Sketch45" against normal blind 5 bodies 1
sketch "Sketch46" plane through (-171.0055, 0.9533, -31.6429) normal (1, 0, 0) x (0, 0, -1)
  line L0 (0, 0) -> (-0.5, 0)
  line L1 (-0.5, 0) -> (-0.5, 11.0833)
  line L2 (-0.5, 11.0833) -> (0, 11.0833)
  line L3 (0, 11.0833) -> (0, 0)
  point P0 (-31.6429, -0.9533)
  dimension "d144" = 0.5
  constraints: 8 end point, 2 parallel, 1 horizontal, 1 perpendicular
  measures "d144" distance of L1.end L2.end
extrude "Extrusion38" add sketch "Sketch46" along normal blind 1 bodies 1
sketch "Sketch47" plane through (-88.0055, 0.9533, -31.6429) normal (-1, 0, 0) x (0, 0, 1)
  line L0 (0, 11) -> (0.5, 11)
  line L1 (0.5, 11) -> (0.5, 0)
  line L2 (0.5, 0) -> (0, 0)
  line L3 (0, 0) -> (0, 11)
  point P0 (31.6429, -0.9533)
  dimension "d147" = 0.5
  constraints: 8 end point, 2 parallel, 1 horizontal, 1 perpendicular
  measures "d147" distance of L1.end L2.end
extrude "Extrusion39" add sketch "Sketch47" along normal blind 1.25 bodies 1
sketch "Sketch48" plane through (-24.7403, 1, -31.6429) normal (1, 0, 0) x (0, 0, -1)
  line L0 (-0.5, -0.0467) -> (0, -0.0467) projected
  line L1 (-0.5, -0.0467) -> (-0.5, 10.9533) projected
  line L2 (0, 10.9533) -> (-0.5, 10.9533) projected
  line L3 (0, 10.9533) -> (0, -0.0467) projected
  point P0 (-31.6429, -1)
extrude "Extrusion40" add sketch "Sketch48" along normal blind 1.25 bodies 1
sketch "Sketch49" plane through (59.2597, 0, -31.6429) normal (0, 0, -1) x (-1, 0, 0)
  line L0 (82.75, 1) -> (82.75, 11.9533) projected
  line L1 (82.75, 11.9533) -> (82.75, 12.2962)
  line L2 (82.75, 12.2962) -> (84, 13)
  line L3 (84, 13) -> (85, 12)
  line L4 (85, 12) -> (84.1938, 11.1938)
  line L5 (84.1938, 11.1938) -> (82.75, 11.8794)
  point P0 (59.2597, 0)
  constraints: 10 end point, 1 perpendicular, 1 point on line, 1 vertical
extrude "Extrusion41" add sketch "Sketch49" against normal up to surface (0.5 mm away) bodies 1
sketch "Sketch50" plane through (59.2597, 0, -31.6429) normal (1, 0, 0) x (0, 0, -1)
  line L0 (-0.5, 12) -> (-0.5, 1) projected
  line L1 (0, 1) -> (-0.5, 1) projected
  line L2 (0, 1) -> (0, 12) projected
  line L3 (-0.5, 12) -> (0, 12) projected
  point P0 (-31.6429, 0)
extrude "Extrusion42" add sketch "Sketch50" against normal blind 2 bodies 1
sketch "Sketch51" plane through (-79.2898, -21, -10.7134) normal (0, 0, 1) x (1, 0, 0)
  circle A0 centre (11, 10.5) radius 2.5 projected
  circle A1 centre (36, 10.5) radius 2.5 projected
  circle A2 centre (11, 10.5) radius 2.6
  circle A3 centre (36, 10.5) radius 2.6
  point P0 (79.2898, 21)
  dimension "d156" = 5.2
  dimension "d157" = 5.2
  constraints: 2 centre point, 2 coincident
  measures "d156" diameter of A2
  measures "d157" diameter of A3
extrude "Extrusion43" cut sketch "Sketch51" against normal blind 5.5 contours A0 | A1 | A3 bodies 1
sketch "Sketch52" plane through (-79.2898, -21, -10.7134) normal (0, 0, 1) x (1, 0, 0)
  circle A0 centre (11, 10.5) radius 2.5 projected
  circle A1 centre (36, 10.5) radius 2.6 projected
  circle A2 centre (11, 10.5) radius 4.6
  circle A3 centre (36, 10.5) radius 4.6
  point P0 (79.2898, 21)
  dimension "d160" = 9.2
  dimension "d161" = 9.2
  constraints: 2 centre point, 2 coincident
  measures "d160" diameter of A2
  measures "d161" diameter of A3
extrude "Extrusion44" cut sketch "Sketch52" against normal blind 2.2 bodies 1
sketch "Sketch53" plane through (59.2597, 0, -31.6429) normal (0, 0, -1) x (-1, 0, 0)
  line L0 (0, 13.5) -> (0, 0) projected
  line L1 (231.2652, 0) -> (0, 0) projected
  line L2 (231.2652, 0) -> (231.2652, 13.5) projected
  line L3 (0, 13.5) -> (231.2652, 13.5) projected
  line L4 (2, 12) -> (2, 1) projected
  line L5 (2, 12) -> (82.75, 12) projected
  line L6 (82.75, 1) -> (82.75, 12) projected
  line L7 (82.75, 1) -> (2, 1) projected
  line L8 (229.2652, 0.9533) -> (148.5152, 0.9533) projected
  line L9 (148.5152, 11.9533) -> (148.5152, 0.9533) projected
  line L10 (148.5152, 11.9533) -> (229.2652, 11.9533) projected
  line L11 (229.2652, 0.9533) -> (229.2652, 11.9533) projected
  point P0 (59.2597, 0)
extrude "Extrusion45" add sketch "Sketch53" along normal blind 6 bodies 1
sketch "Sketch54" plane through (57.2597, 12, -31.1429) normal (0, 0, 1) x (1, 0, 0)
  line L0 (1, 0) -> (1, -11) projected
  line L1 (0, 0) -> (1, 0) projected
  line L2 (0, -11) -> (0, 0) projected
  line L3 (1, -11) -> (0, -11) projected
  point P0 (-57.2597, -12)
extrude "Extrusion46" cut sketch "Sketch54" against normal blind 6 bodies 1
sketch "Sketch55" plane through (-24.7403, 1, -31.1429) normal (0, 0, 1) x (1, 0, 0)
  line L0 (0, 0) -> (0, 11) projected
  line L1 (1.25, 0) -> (0, 0) projected
  line L2 (1.25, 11) -> (1.25, 0) projected
  line L3 (0, 11) -> (1.25, 11) projected
  point P0 (24.7403, -1)
extrude "Extrusion47" cut sketch "Sketch55" against normal blind 6 bodies 1
sketch "Sketch56" plane through (58.2597, 1, -28) normal (0, 0, -1) x (-1, 0, 0)
  line L0 (0, 0) -> (0, 11) projected
  line L1 (4, 0) -> (0, 0) projected
  line L2 (4, 11) -> (4, 0) projected
  line L3 (0, 11) -> (4, 11) projected
  point P0 (58.2597, -1)
extrude "Extrusion48" add sketch "Sketch56" along normal blind 6 bodies 1
sketch "Sketch57" plane through (1.2597, 12, -28) normal (0, 0, -1) x (-1, 0, 0)
  line L0 (26, -11) -> (0, -11) projected
  line L1 (26, -11) -> (26, 0) projected
  line L2 (0, 0) -> (26, 0) projected
  line L3 (0, 0) -> (0, -11) projected
  point P0 (1.2597, -12)
extrude "Extrusion49" add sketch "Sketch57" along normal blind 6 bodies 1
sketch "Sketch58" plane through (-88.0055, 0.9533, -31.1429) normal (0, 0, 1) x (1, 0, 0)
  line L0 (0, 11) -> (0, 0) projected
  line L1 (-1.25, 11) -> (0, 11) projected
  line L2 (-1.25, 0) -> (-1.25, 11) projected
  line L3 (0, 0) -> (-1.25, 0) projected
  point P0 (88.0055, -0.9533)
extrude "Extrusion50" cut sketch "Sketch58" against normal blind 6 bodies 1
sketch "Sketch59" plane through (-171.0055, 0.9533, -31.1429) normal (0, 0, 1) x (1, 0, 0)
  line L0 (0, 11) -> (1, 11) projected
  line L1 (0, 0) -> (0, 11) projected
  line L2 (1, 0) -> (0, 0) projected
  line L3 (1, 11) -> (1, 0) projected
  point P0 (171.0055, -0.9533)
extrude "Extrusion51" cut sketch "Sketch59" against normal blind 6 bodies 1
sketch "Sketch60" plane through (-167.0055, 11.9533, -28) normal (0, 0, -1) x (-1, 0, 0)
  line L0 (4, 0) -> (4, -11) projected
  line L1 (0, 0) -> (4, 0) projected
  line L2 (0, -11) -> (0, 0) projected
  line L3 (4, -11) -> (0, -11) projected
  point P0 (-167.0055, -11.9533)
extrude "Extrusion52" add sketch "Sketch60" along normal blind 6 bodies 1
sketch "Sketch61" plane through (1.2597, 12, -28) normal (0, 0, -1) x (-1, 0, 0)
  line L0 (89.2652, -0.0467) -> (115.2652, -0.0467) projected
  line L1 (89.2652, -0.0467) -> (89.2652, -11.0467) projected
  line L2 (115.2652, -11.0467) -> (89.2652, -11.0467) projected
  line L3 (115.2652, -11.0467) -> (115.2652, -0.0467) projected
  point P0 (1.2597, -12)
extrude "Extrusion53" add sketch "Sketch61" along normal blind 6 bodies 1
sketch "Sketch62" plane through (59.2597, 0, -37.6429) normal (0, 0, -1) x (-1, 0, 0)
  point P0 (59.2597, 0)
sketch "Sketch63" plane through (-89.2555, 0.9533, -31.6429) normal (-1, 0, 0) x (0, 0, 1)
  line L0 (-5.5, 0) -> (-5.5, 11) projected
  line L1 (-6, 11) -> (-5.5, 11) projected
  line L2 (-6, 0) -> (-6, 11) projected
  line L3 (-5.5, 0) -> (-6, 0) projected
  point P0 (31.6429, -0.9533)
extrude "Extrusion54" add sketch "Sketch63" along normal blind 1 bodies 1
sketch "Sketch64" plane through (-23.4903, 1, -31.6429) normal (1, 0, 0) x (0, 0, -1)
  line L0 (5.5, 11) -> (5.5, 0) projected
  line L1 (6, 0) -> (5.5, 0) projected
  line L2 (6, 11) -> (6, 0) projected
  line L3 (5.5, 11) -> (6, 11) projected
  point P0 (-31.6429, -1)
extrude "Extrusion55" add sketch "Sketch64" along normal blind 1 bodies 1
sketch "Sketch65" plane through (-56.3729, 3.5, -21.8037) normal (0, -1, 0) x (1, 0, 0)
  circle A0 centre (0, 0) radius 6.1 projected
  circle A1 centre (0, 0) radius 3.0578 projected
  point P0 (56.3729, 21.8037)
extrude "Extrusion56" cut sketch "Sketch65" against normal blind 3 bodies 1
sketch "Sketch66" plane through (-56.3729, 6.5, -21.8037) normal (0, -1, 0) x (1, 0, 0)
  circle A0 centre (0, 0) radius 6.1 projected
  circle A1 centre (0, 0) radius 3.0578 projected
  point P0 (56.3729, 21.8037)
extrude "Extrusion57" add sketch "Sketch66" along normal blind 1.3 bodies 1
equation "\"d56\" = d63"
equation "\"d57\" = 0.160083 * Sketch17_Pitch"
equation "\"d58\" = 0.160083 * Sketch17_Pitch"
equation "\"d61\" = Sketch17_Pitch"
equation "\"d74\" = d81"
equation "\"d75\" = 0.160083 * Sketch19_Pitch"
equation "\"d76\" = 0.160083 * Sketch19_Pitch"
equation "\"d79\" = Sketch19_Pitch"
equation "\"d63\" = 55deg"
equation "\"Sketch17_Pitch\" = 0.8"
equation "\"d81\" = 55deg"
equation "\"Sketch19_Pitch\" = 0.8"
body "Solid1"
body "Solid2"
body "Solid3"
